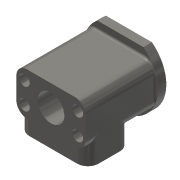
# Autodesk Inventor part: valvebody
Saved by Autodesk Inventor 2022 Beta2 (Build 260130000, 130) ContinuousBuild 0
## iProperties
Shininess: 64.0
Length Units: 11272
Angle Units: 11279
Time Units: 11290
Mass Units: 11286
Length Display Precision: 3
Angle Display Precision: 2
Created: 2002-02-11
Part Number: valvebody
Document SubType Name: Modeling
Designer: Administrator
Density: 1 g/cm^3
Material: Generic
Appearance: Steel - Cast
Density: 0.0
Volumn: 0.0
Area: 0.0
PropertySet Name: Model Information
Control State: 0
Master: False
Checked Out: False
Author: Administrator
Autodesk Inventor part; units mm, degrees
ref_plane "YZ Plane" through (0, 0, 0) normal (1, 0, 0) x (0, 1, 0)
sketch "Sketch1" plane through (0, 0, 0) normal (0, 0, 1) x (1, 0, 0)
  line L0 (-29.1534, 12.578) -> (25.5151, 12.578)
  arc A0 (-29.1534, 12.578) -> (25.5151, 12.578) centre (-1.8191, -22.474) ccw
  dimension "d0" = 44.45
  dimension "d1" = 35.052
  constraints: 2 end point, 2 point on circle, 1 centre point, 1 horizontal
  measures "d0" radius of A0
  measures "d1" distance from line of L0 A0.centre
extrude "Extrusion1" add sketch "Sketch1" along normal blind 10.16
sketch "Sketch2" plane through (0, 0, 10.16) normal (0, 0, 1) x (1, 0, 0)
  arc A0 (-29.1534, 12.578) -> (25.5151, 12.578) centre (-1.8191, -22.474) ccw projected
  line L0 (-43.0941, 2.926) -> (39.4559, 2.926)
  line L1 (39.4559, 2.926) -> (39.4559, -47.874)
  line L2 (39.4559, -47.874) -> (-43.0941, -47.874)
  line L3 (-43.0941, -47.874) -> (-43.0941, 2.926)
  circle A1 centre (-1.8191, -22.474) radius 41.275 construction
  circle A2 centre (-1.8191, -22.474) radius 25.4 construction
  dimension "d4" = 82.55
  dimension "d5" = 50.8
  constraints: 8 end point, 4 tangent, 2 centre point, 2 coincident, 2 parallel, 1 concentric, 1 horizontal, 1 perpendicular
  measures "d4" distance of L1.end L2.end
  measures "d5" distance of L2.end L0.start
extrude "Extrusion2" add sketch "Sketch2" along normal blind 82.55 contours L0 A0 L1 L2 L3 | A0 L3 L0 | L0 L1 A0 | A0 L2 L3 | L1 L2 A0
fillet "Fillet1" radius 12.7 4 edges at (-43.0941, -47.874, 51.435) (-43.0941, 2.926, 51.435) (39.4559, -47.874, 51.435) (39.4559, 2.926, 51.435)
ref_plane "Work Plane1" through (-30.3941, -66.924, 10.16) normal (0, -1, 0) x (1, 0, 0)
sketch "Sketch3" plane through (-30.3941, -66.924, 10.16) normal (0, -1, 0) x (1, 0, 0)
  line L0 (-12.7, 80.01) -> (69.85, 80.01)
  line L1 (69.85, 80.01) -> (69.85, 29.21)
  line L2 (69.85, 29.21) -> (-12.7, 29.21)
  line L3 (-12.7, 29.21) -> (-12.7, 80.01)
  line L4 (-12.7, 82.55) -> (-12.7, 0) projected
  line L5 (69.85, 0) -> (69.85, 82.55) projected
  dimension "d11" = 50.8
  constraints: 8 end point, 2 collinear, 2 parallel, 1 horizontal, 1 perpendicular
  measures "d11" distance of L2.end L0.start
extrude "Extrusion3" add sketch "Sketch3" against normal up to next
fillet "Fillet2" radius 12.7 4 edges at (-43.0941, -51.049, 90.17) (-43.0941, -51.049, 39.37) (39.4559, -51.049, 39.37) (39.4559, -51.049, 90.17)
sketch "Sketch4" plane through (0, 0, 92.71) normal (0, 0, 1) x (1, 0, 0)
  line L0 (-43.0941, -35.174) -> (-43.0941, -9.774) projected
  line L1 (26.7559, -47.874) -> (-30.3941, -47.874) projected
  line L2 (39.4559, -9.774) -> (39.4559, -35.174) projected
  line L3 (-30.3941, 2.926) -> (26.7559, 2.926) projected
  line L4 (-33.5691, -9.774) -> (29.9309, -9.774)
  line L5 (29.9309, -9.774) -> (29.9309, -35.174)
  line L6 (29.9309, -35.174) -> (-33.5691, -35.174)
  line L7 (-33.5691, -35.174) -> (-33.5691, -9.774)
  circle A0 centre (-1.8191, -22.474) radius 12.7 construction
  circle A1 centre (-1.8191, -22.474) radius 41.275 construction
  circle A2 centre (-1.8191, -22.474) radius 31.75 construction
  circle A3 centre (-1.8191, -22.474) radius 25.4 construction
  dimension "d15" = 63.5
  dimension "d16" = 25.4
  constraints: 8 end point, 8 tangent, 4 centre point, 3 coincident, 2 parallel, 1 horizontal, 1 perpendicular
  measures "d15" distance of L5.end L6.end
  measures "d16" distance of L6.end L4.start
hole "Hole1" at (-33.5691, -9.774, 92.71) at (-33.5691, -35.174, 92.71) at (29.9309, -35.174, 92.71) at (29.9309, -9.774, 92.71) direction (0, 0, -1) diameter 12.7 end through all
sketch "Sketch5" plane through (0, 0, 92.71) normal (0, 0, 1) x (1, 0, 0)
  line L0 (-43.0941, -35.174) -> (-43.0941, -9.774) projected
  line L1 (26.7559, -47.874) -> (-30.3941, -47.874) projected
  line L2 (39.4559, -9.774) -> (39.4559, -35.174) projected
  line L3 (-30.3941, 2.926) -> (26.7559, 2.926) projected
  circle A0 centre (-1.8191, -22.474) radius 41.275 construction
  circle A1 centre (-1.8191, -22.474) radius 25.4 construction
  constraints: 4 tangent, 2 centre point, 2 coincident
hole "Hole2" at (-1.8191, -22.474, 92.71) direction (0, 0, -1) diameter 31.75 end through all
sketch "Sketch6" plane through (-30.3941, -66.924, 10.16) normal (0, -1, 0) x (1, 0, 0)
  arc A0 (57.15, 29.21) -> (69.85, 41.91) centre (57.15, 41.91) ccw projected
  line L0 (69.85, 67.31) -> (69.85, 41.91) projected
  line L1 (0, 80.01) -> (57.15, 80.01) projected
  arc A1 (0, 80.01) -> (-12.7, 67.31) centre (0, 67.31) ccw projected
  line L2 (-12.7, 41.91) -> (-12.7, 67.31) projected
  line L3 (57.15, 29.21) -> (0, 29.21) projected
  line L4 (0, 67.31) -> (57.15, 67.31)
  line L5 (57.15, 67.31) -> (57.15, 41.91)
  line L6 (57.15, 41.91) -> (0, 41.91)
  line L7 (0, 41.91) -> (0, 67.31)
  circle A2 centre (28.575, 54.61) radius 28.575 construction
  circle A3 centre (28.575, 54.61) radius 12.7 construction
  circle A4 centre (28.575, 54.61) radius 41.275 construction
  circle A5 centre (28.575, 54.61) radius 25.4 construction
  dimension "d31" = 25.4
  dimension "d32" = 57.15
  constraints: 8 end point, 8 tangent, 4 centre point, 3 coincident, 2 parallel, 1 horizontal, 1 perpendicular
  measures "d31" distance of L6.end L4.start
  measures "d32" distance of L5.end L6.end
hole "Hole3" at (-30.3941, -66.924, 77.47) at (-30.3941, -66.924, 52.07) at (26.7559, -66.924, 52.07) at (26.7559, -66.924, 77.47) direction (0, 1, 0) diameter 7.7978 depth 31.75 tip angle 118 thread size "3/8-16 UNC" class "1B" standard "ANSI Unified Screw Threads"
sketch "Sketch7" plane through (-30.3941, -66.924, 10.16) normal (0, -1, 0) x (1, 0, 0)
  line L0 (69.85, 67.31) -> (69.85, 41.91) projected
  line L1 (0, 80.01) -> (57.15, 80.01) projected
  line L2 (-12.7, 41.91) -> (-12.7, 67.31) projected
  line L3 (57.15, 29.21) -> (0, 29.21) projected
  circle A0 centre (28.575, 54.61) radius 41.275 construction
  circle A1 centre (28.575, 54.61) radius 25.4 construction
  constraints: 4 tangent, 2 centre point, 2 coincident
hole "Hole4" at (-1.8191, -66.924, 64.77) direction (0, 1, 0) diameter 31.75 depth 25.4 tip angle 118
ref_plane "Work Plane2" through (-1.8191, -54.224, 64.77) normal (0, 0, 1) x (1, 0, 0)
sketch "Sketch8" plane through (-1.8191, -54.224, 64.77) normal (0, 0, 1) x (1, 0, 0)
  circle A0 centre (0, 31.75) radius 22.225
  circle A1 centre (0, 31.75) radius 15.875 projected
  dimension "d48" = 44.45
  constraints: 1 centre point, 1 concentric
  measures "d48" diameter of A0
extrude "Extrusion4" cut sketch "Sketch8" against normal mid plane 12.7
fillet "Fillet3" radius 2.54 14 edges at (-1.8191, -47.874, 10.16) (-39.3744, -44.1543, 10.16) (-43.0941, -22.474, 10.16) (-39.3744, -0.7938, 10.16) (-1.8191, 2.926, 10.16) (35.7361, -0.7938, 10.16) (39.4559, -22.474, 10.16) (35.7361, -44.1543, 10.16) (-1.8191, -47.874, 90.17) (35.7361, -44.1543, 86.4503) (-39.3744, -44.1543, 86.4503) (35.7361, -44.1543, 43.0897) (-1.8191, -47.874, 39.37) (-39.3744, -44.1543, 43.0897)
body "Solid1"
